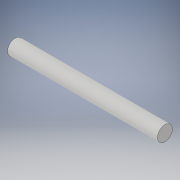
# Autodesk Inventor part: pin
Saved by Autodesk Inventor 2018 (Build 220112000, 112)
## iProperties
Created: 2021-03-17
Part Number: pin
Material: Generic
Document SubType Name: Modeling
Designer: Jyoti Soni
Density: 1 g/cm^3
Appearance: Default
Author: Jyoti Soni
Autodesk Inventor part; units mm, degrees
ref_plane "YZ Plane" through (0, 0, 0) normal (1, 0, 0) x (0, 1, 0)
ref_plane "XZ Plane" through (0, 0, 0) normal (0, 1, 0) x (-1, 0, 0)
ref_plane "XY Plane" through (0, 0, 0) normal (0, 0, 1) x (1, 0, 0)
sketch "Sketch1" plane through (0, 0, 0) normal (0, 0, 1) x (1, 0, 0)
  point P0 (0, 0)
sketch "Sketch2" plane through (0, 0, 0) normal (0, 0, 1) x (1, 0, 0)
  line L0 (0, 0) -> (35, 0)
  line L1 (35, 0) -> (35, 1.75)
  line L2 (35, 1.75) -> (0, 1.75)
  line L3 (0, 1.75) -> (0, 0)
  dimension "d0" = 1.75
  dimension "d1" = 35
  constraints: 8 end point, 2 parallel, 1 horizontal, 1 perpendicular
  measures "d0" distance of L2.end L0.start
  measures "d1" distance of L1.end L2.end
revolve "Revolution1" add sketch "Sketch2" angle 360 about axis through (0, 0, 0) along (1, 0, 0)
body "Solid1"
